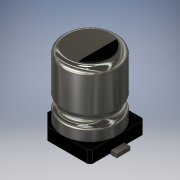
# Autodesk Inventor part: SMTElectro4x4x6_5
Saved by Autodesk Inventor 2016 (Build 200138000, 138)
## iProperties
Created: 2016-08-10
Part Number: SMTElectro4x4x6_5
Material: Generic
Document SubType Name: Modeling
Designer: jfixelle
Density: 1 g/cm^3
Appearance: Gray
Author: jfixelle
Autodesk Inventor part; units mm, degrees
ref_plane "YZ Plane" through (0, 0, 0) normal (1, 0, 0) x (0, 1, 0)
ref_plane "XZ Plane" through (0, 0, 0) normal (0, 1, 0) x (-1, 0, 0)
ref_plane "XY Plane" through (0, 0, 0) normal (0, 0, 1) x (1, 0, 0)
sketch "Sketch1" plane through (0, 0, 0) normal (0, 1, 0) x (-1, 0, 0)
  line L0 (2.25, 2.25) -> (-2.25, 2.25)
  line L1 (-2.25, 2.25) -> (-2.25, -2.25)
  line L2 (-2.25, -2.25) -> (2.25, -2.25)
  line L3 (2.25, -2.25) -> (2.25, 2.25)
  line L4 (2.25, 1.25) -> (1.25, 2.25)
  line L5 (2.25, -1.25) -> (1.25, -2.25)
  point P0 (0, 0)
  dimension "d0" = 4.5
  dimension "d1" = 4.5
  dimension "d2" = 2.25
  dimension "d3" = 2.25
  dimension "d4" = 45
  dimension "d5" = 45
  dimension "d6" = 1
  dimension "d7" = 1
  constraints: 12 end point, 4 point on line, 2 parallel, 1 horizontal, 1 perpendicular
  measures "d0" distance of L0.end L1.end
  measures "d1" distance of L1.end L2.end
  measures "d2" distance from line of L2 point (0, 0)
  measures "d3" distance from line of L1 point (0, 0)
  measures "d4" angle of L3 L5
  measures "d5" angle of L3 L4
  measures "d6" distance from line of L3 L4.end
  measures "d7" distance from line of L3 L5.end
extrude "Extrusion1" add sketch "Sketch1" along normal blind 1 contours L4 L3 L5 L2 L1 L0
chamfer "Chamfer1" distance 0.2 angle 45 2 edges at (2.25, 0.5, 2.25) (2.25, 0.5, -2.25)
sketch "Sketch2" plane through (0, 1, 0) normal (0, 1, 0) x (1, 0, 0)
  circle A0 centre (0, 0) radius 2.25
  dimension "d13" = 4.5
  constraints: 1 centre point, 1 coincident
  measures "d13" diameter of A0
extrude "Extrusion2" add sketch "Sketch2" along normal blind 5.2
sketch "Sketch3" plane through (0, 0, 0) normal (0, -1, 0) x (1, 0, 0)
  line L0 (-2.25, 0.55) -> (-2.25, -0.55)
  line L1 (-2.75, -0.55) -> (-2.75, 0.55)
  line L2 (-2.75, 0.55) -> (-2.25, 0.55)
  line L3 (-2.75, -0.55) -> (-2.25, -0.55)
  point P0 (0, 0)
  dimension "d16" = 1.1
  dimension "d18" = 2.25
  dimension "d33" = 2.75
  constraints: 8 end point, 2 parallel, 1 horizontal
  measures "d16" distance of L1.start L1.end
  measures "d18" distance from line of point (0, 0) L0
  measures "d33" distance from line of point (0, 0) L1
extrude "Extrusion3" add sketch "Sketch3" along normal blind 0.1 and the other way blind 0.2
mirror "Mirror1" about plane through (0, 0, 0) normal (1, 0, 0) of "Extrusion3"
fillet "Fillet1" radius 0.5 1 edges at (-2.25, 6.2, 0)
sketch "Sketch4" plane through (0, 6.2, 0) normal (0, 1, 0) x (1, 0, 0)
  circle A0 centre (0, 0) radius 6.25
  circle A1 centre (0, 0) radius 2.25 projected
  line L0 (3.2451, -4.6893) -> (3.2427, 4.6909)
  arc A2 (3.2451, -4.6893) -> (3.2427, 4.6909) centre (0, 0) ccw
  arc A3 (0.6558, -1.5332) -> (0.6558, 1.5332) centre (0, 0) ccw
  line L1 (0.6558, -1.5332) -> (0.6558, 1.5332)
  constraints: 4 end point, 4 point on circle, 3 centre point, 3 coincident, 1 vertical
extrude "Extrusion5" add sketch "Sketch4" along normal blind 0.1 contours L1 A3
sketch "Sketch5" plane through (0, 0, 0) normal (0, 0, 1) x (1, 0, 0)
  line L0 (2.25, 1) -> (2.25, 5.7) projected
  line L1 (0, -1.3032) -> (0, 7.8193) projected
  circle A0 centre (2.25, 2.3529) radius 0.4103
  point P0 (0, 0)
  constraints: 1 centre point, 1 point on line
revolve "Revolution1" cut sketch "Sketch5" angle 360 about axis through (0, -10, 0) along (0, 1, 0)
fillet "Fillet4" radius 0.2 2 edges at (-2.25, 1.9426, 0) (-2.25, 2.7632, 0)
body "Solid1"
